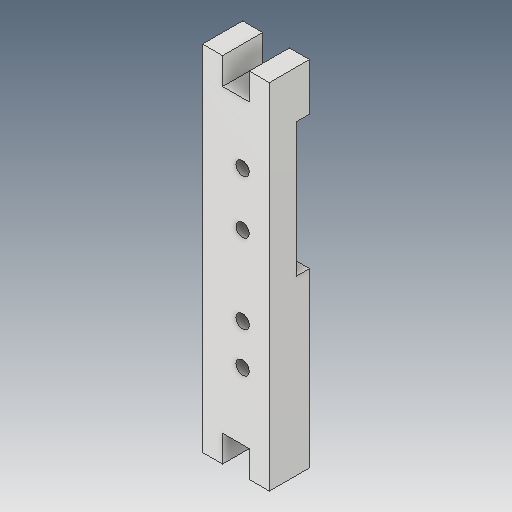
# Autodesk Inventor part: CP002
Saved by Autodesk Inventor 2017 (Build 210142000, 142)
## iProperties
Created: 2017-05-15
Part Number: CP002
Material: ABS Plastic
Document SubType Name: Modeling
Designer: zallen
Density: 1.06 g/cm^3
Appearance: Smooth - White
Mass: 43.0637 g
Surface Area: 123.613 cm^2
Volume: 40.6261 cm^3
Author: zallen
Autodesk Inventor part; units mm, degrees
ref_plane "YZ Plane" through (0, 0, 0) normal (1, 0, 0) x (0, 1, 0)
ref_plane "XZ Plane" through (0, 0, 0) normal (0, 1, 0) x (-1, 0, 0)
ref_plane "XY Plane" through (0, 0, 0) normal (0, 0, 1) x (1, 0, 0)
sketch "Sketch1" plane through (0, 0, 0) normal (0, 0, 1) x (1, 0, 0)
  circle A0 centre (-175, 0) radius 225 construction
  circle A1 centre (-175, 0) radius 200 construction
  line L0 (-25, 0) -> (-25, -132.2876)
  line L1 (-17.5, 0) -> (-17.5, -10)
  line L2 (-17.5, -10) -> (-7.5, -10)
  line L3 (-17.5, -10) -> (-7.5, -10) construction
  line L4 (-7.5, -10) -> (-7.5, 0)
  line L5 (-25, 0) -> (-17.5, 0)
  line L6 (-7.5, 0) -> (0, 0)
  line L7 (0, 0) -> (0, -132.2876)
  line L8 (-17.5, -132.2876) -> (-17.5, -122.2876)
  line L9 (-17.5, -132.2876) -> (-7.5, -132.2876) construction
  line L10 (-17.5, -122.2876) -> (-7.5, -122.2876)
  line L11 (-7.5, -122.2876) -> (-7.5, -132.2876)
  line L12 (-25, -132.2876) -> (-17.5, -132.2876)
  line L13 (-7.5, -132.2876) -> (0, -132.2876)
  dimension "d0" = 450
  dimension "d1" = 25
  dimension "d2" = 175
  dimension "d3" = 25
  dimension "d5" = 10
  dimension "d6" = 10
  dimension "d7" = 0
  dimension "d8" = 7.5
  dimension "d11" = 10
  dimension "d12" = 90
  dimension "d13" = 10
  dimension "d14" = 90
  constraints: 28 end point, 5 horizontal, 3 vertical, 2 equal length, 1 centre point, 1 perpendicular, 3 other
  measures "d0" diameter of A0
  measures "d2" distance of A0.centre L6.end
  measures "d3" distance of L6.end L0.start
  measures "d5" distance of L1.start L1.end
  measures "d6" distance of L1.end L2.end
  measures "d7" distance between parallel lines of L2 L3
  measures "d8" distance of L0.start L1.start
  measures "d11" distance of L8.start L8.end
  measures "d12" angle of L9 L8
  measures "d13" distance of L8.end L10.end
  measures "d14" angle of L8 L10
extrude "Extrusion1" add sketch "Sketch1" along normal blind 15
sketch "Sketch2" plane through (0, 0, 15) normal (0, 0, 1) x (1, 0, 0)
  line L0 (0, -17.7124) -> (-20, -17.7124) construction
  line L1 (-20, -17.7124) -> (-20, -67.7124) construction
  line L2 (-20, -67.7124) -> (0, -67.7124) construction
  line L3 (0, -67.7124) -> (0, -17.7124) construction
  line L4 (-7.5, -132.2876) -> (0, -132.2876) construction
  circle A0 centre (-10, -32.7124) radius 2.5
  circle A1 centre (-10, -52.7124) radius 2.5
  point P0 (0, 0)
  dimension "d15" = 20
  dimension "d16" = 50
  dimension "d17" = 64.5751
  dimension "d18" = 5
  dimension "d19" = 5
  dimension "d20" = 15
  dimension "d21" = 15
  dimension "d22" = 10
  dimension "d23" = 10
  constraints: 8 end point, 2 centre point, 2 parallel, 1 horizontal, 1 perpendicular
  measures "d15" distance of L2.end L1.end
  measures "d16" distance of L1.end L0.end
  measures "d17" distance between parallel lines of L4 L2
  measures "d18" diameter of A0
  measures "d19" diameter of A1
  measures "d20" distance from line of L0 A0.centre
  measures "d21" distance from line of L2 A1.centre
  measures "d22" distance from line of L3 A0.centre
  measures "d23" distance from line of L3 A1.centre
extrude "Extrusion2" cut sketch "Sketch2" against normal through all
thread "Thread1" size "M5x0.8" class "6H" standard "ANSI Metric M Profile" full length
thread "Thread2" size "M5x0.8" class "6H" standard "ANSI Metric M Profile" full length
sketch "Sketch3" plane through (0, 0, 15) normal (0, 0, 1) x (1, 0, 0)
  circle A0 centre (-10, -82.2876) radius 2.5
  circle A1 centre (-10, -97.2876) radius 2.5
  line L0 (0, -132.2876) -> (0, 0) projected
  line L1 (-7.5, -132.2876) -> (0, -132.2876) projected
  dimension "d30" = 5
  dimension "d31" = 5
  dimension "d32" = 10
  dimension "d33" = 10
  dimension "d34" = 15
  dimension "d35" = 35
  constraints: 2 centre point
  measures "d30" diameter of A0
  measures "d31" diameter of A1
  measures "d32" distance from line of L0 A0.centre
  measures "d33" distance from line of L0 A1.centre
  measures "d34" distance of A1.centre A0.centre
  measures "d35" distance from line of A1.centre L1
extrude "Extrusion3" cut sketch "Sketch3" against normal through all
thread "Thread3" size "M5x0.8" class "6H" standard "ANSI Metric M Profile" full length
thread "Thread4" size "M5x0.8" class "6H" standard "ANSI Metric M Profile" full length
sketch "Sketch5" plane through (0, 0, 0) normal (0, 0, -1) x (-1, 0, 0)
  line L0 (0, -17.7124) -> (20, -17.7124)
  line L1 (20, -17.7124) -> (20, -67.7124)
  line L2 (20, -67.7124) -> (0, -67.7124)
  line L3 (0, -67.7124) -> (0, -17.7124)
  point P0 (0, 0)
  dimension "d50" = 20
  dimension "d51" = 50
  dimension "d52" = 17.7124
  constraints: 8 end point, 2 parallel, 1 horizontal, 1 perpendicular
  measures "d50" distance of L1.end L2.end
  measures "d51" distance of L0.end L1.end
  measures "d52" distance of point (0, 0) L0.start
extrude "Extrusion5" cut sketch "Sketch5" against normal blind 5
body "Solid1"
